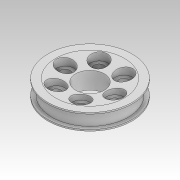
# Autodesk Inventor part: J3DriveGear
Saved by Autodesk Inventor 2020 (Build 240168000, 168)
## iProperties
Created: 2021-11-27
Part Number: J3DriveGear
Material: Generic
Document SubType Name: Modeling
Designer: DDeGo
Density: 1 g/cm^3
Appearance: Default
Author: DDeGo
Autodesk Inventor part; units mm, degrees
ref_plane "YZ Plane" through (0, 0, 0) normal (1, 0, 0) x (0, 1, 0)
ref_plane "XZ Plane" through (0, 0, 0) normal (0, 1, 0) x (-1, 0, 0)
ref_plane "XY Plane" through (0, 0, 0) normal (0, 0, 1) x (1, 0, 0)
sketch "Sketch1" plane through (0, 0, 0) normal (0, 0, 1) x (1, 0, 0)
  line L0 (0, 9) -> (0, 0) construction
  line L1 (0, 0) -> (7.5, 0) construction
  line L2 (17.45, 0) -> (17.45, 1.5)
  line L3 (17.45, 1.5) -> (18.95, 1.5)
  line L4 (22, 3) -> (20, 3)
  line L5 (20, 3) -> (20, 10)
  line L6 (20, 10) -> (22, 10)
  line L7 (22, 10) -> (22, 10.75)
  line L8 (18.95, 1.5) -> (22, 2.25)
  line L9 (22, 2.25) -> (22, 3)
  line L10 (7.5, 9) -> (18, 10.75)
  line L11 (18, 10.75) -> (22, 10.75)
  line L12 (7.5, 9) -> (7.5, 0)
  line L13 (7.5, 0) -> (17.45, 0)
  dimension "d0" = 7
  dimension "d1" = 17.45
  dimension "d2" = 1.5
  dimension "d3" = 1.5
  dimension "d4" = 1.5
  dimension "d5" = 2
  dimension "d6" = 0.75
  dimension "d7" = 20
  dimension "d8" = 0.75
  dimension "d11" = 2
  dimension "d27" = 7.5
  dimension "d28" = 9
  constraints: 28 end point, 11 perpendicular, 2 parallel, 1 collinear, 1 horizontal, 1 vertical
  measures "d0" distance of L4.end L5.end
  measures "d1" distance between parallel lines of L0 L2
  measures "d2" distance of L2.start L2.end
  measures "d3" distance of L2.end L3.end
  measures "d4" distance between parallel lines of L3 L4
  measures "d5" distance of L4.start L4.end
  measures "d6" distance of L8.end L4.start
  measures "d7" distance between parallel lines of L0 L5
  measures "d8" distance of L6.end L7.end
  measures "d11" distance from line of L10.end L5
  measures "d27" distance between parallel lines of L0 L12
  measures "d28" distance of L10.start L1.end
revolve "Revolution1" add sketch "Sketch1" angle 360 about axis through (0, 9, 0) along (0, -1, 0)
sketch "Sketch2" plane through (0, 0, 0) normal (0, -1, 0) x (1, 0, 0)
  line L0 (0, 0) -> (13, 0) construction
  circle A0 centre (13, 0) radius 2.55
  circle A1 centre (6.5, 11.2583) radius 2.55
  circle A2 centre (-6.5, 11.2583) radius 2.55
  circle A3 centre (-13, 0) radius 2.55
  circle A4 centre (-6.5, -11.2583) radius 2.55
  circle A5 centre (6.5, -11.2583) radius 2.55
  dimension "d15" = 5.1
  dimension "d16" = 13
  dimension "d19" = 360
  constraints: 6 centre point, 2 end point, 1 coincident, 1 horizontal, 13 other
  measures "d15" diameter of A0
  measures "d16" distance of L0.start L0.end
extrude "Extrusion1" cut sketch "Sketch2" against normal through all
ref_plane "Work Plane1" through (0, 6.5, 0) normal (0, -1, 0) x (1, 0, 0)
sketch "Sketch3" plane through (0, 6.5, 0) normal (0, -1, 0) x (1, 0, 0)
  circle A0 centre (-6.5, 11.2583) radius 2.55 projected
  circle A1 centre (-13, 0) radius 2.55 projected
  circle A2 centre (-6.5, -11.2583) radius 2.55 projected
  circle A3 centre (-6.5, 11.2583) radius 2.55 projected
  circle A4 centre (6.5, 11.2583) radius 2.55 projected
  circle A5 centre (13, 0) radius 2.55 projected
  circle A6 centre (6.5, -11.2583) radius 2.55 projected
  circle A7 centre (0, 0) radius 17.45 projected
  circle A8 centre (6.5, 11.2583) radius 4.5
  circle A9 centre (-6.5, 11.2583) radius 4.5
  circle A10 centre (-13, 0) radius 4.5
  circle A11 centre (-6.5, -11.2583) radius 4.5
  circle A12 centre (6.5, -11.2583) radius 4.5
  circle A13 centre (13, 0) radius 4.5
  dimension "d24" = 9
  constraints: 6 centre point, 6 coincident, 5 equal radius
  measures "d24" diameter of A9
extrude "Extrusion2" cut sketch "Sketch3" against normal through all contours A0 | A1 | A2 | A4 | A5 | A6 | A7 A13 | A7 A13 | A8 A7 | A7 A8 | A12 A7 | A7 A12 | A9 A7 | A7 A9 | A11 A7 | A7 A11 | A10 A7 | A7 A10
equation "\"d8\" = d6"
body "Solid1"
